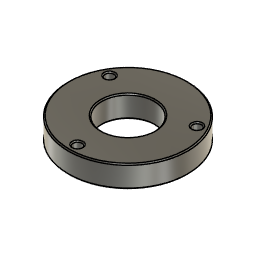
binocular_spacer v1 (Autodesk Fusion 360 design; units mm, degrees)
Autodesk Fusion 360 part; units mm, degrees
sketch "Sketch1" plane through (0, 0, 0) normal (0, 0, 1) x (1, 0, 0)
  circle A0 centre (0, 0) radius 27.25
  circle A1 centre (0, 0) radius 12
  line L0 (0, -27.25) -> (0, -25.05)
  circle A2 centre (0, -23.05) radius 2
  circle A3 centre (19.9619, 11.525) radius 2
  circle A4 centre (-19.9619, 11.525) radius 2
  dimension "d1" = 54.5
  dimension "d2" = 24
  dimension "d5" = 2.2
  dimension "d6" = 4
  dimension "d8" = 360
  constraint coincident A0.centre A1.centre
  constraint vertical L0
  constraint coincident A0 L0.start
  constraint coincident L0.end A2
  measures "d1" diameter of A0
  measures "d2" diameter of A1
  measures "d5" distance of L0.start L0.end
  measures "d6" diameter of A2
extrude "Extrude1" add sketch "Sketch1" along normal blind 10
chamfer "Chamfer1" distance 0.5 angle 45 2 faces at (-19.6319, 4.2187, 10) (-19.6319, 4.2187, 0)
